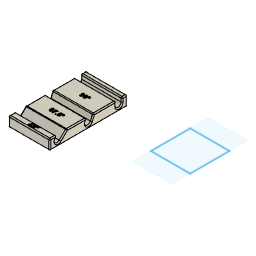
boulderStand v3 (Autodesk Fusion 360 design; units mm, degrees)
Autodesk Fusion 360 part; units mm, degrees
(part 1 of 3)
sketch "Sketch1" plane through (0, 0, 0) normal (0, 0, 1) x (1, 0, 0)
  line L0 (0, 0) -> (80, 0)
  line L1 (80, 0) -> (80, 150)
  line L2 (80, 150) -> (0, 150)
  line L3 (0, 150) -> (0, 0)
  dimension "d1" = 80
  dimension "d2" = 150
  constraint horizontal L0
  constraint vertical L1
  constraint horizontal L2
  constraint vertical L3
  constraint coincident L0.start L3.end
  measures "d1" distance of L0.start L0.end
  measures "d2" distance of L0.start L2.end
extrude "Extrude1" add sketch "Sketch1" along normal blind 20
sketch "Sketch2" plane through (0, 0, 0) normal (-1, 0, 0) x (0, -1, 0)
  line L0 (-150, 0) -> (0, 0)
  line L1 (0, 0) -> (0, 20)
  line L2 (0, 20) -> (-150, 20)
  line L3 (-150, 20) -> (-150, 0)
  line L4 (-140, 10) -> (-134, 10)
  arc A0 (-139.9709, 11.6408) -> (-127.9709, 11.6408) centre (-133.9709, 11.6408) ccw
  line L5 (-139.9709, 11.6408) -> (-139.9709, 20)
  line L6 (-127.9709, 11.6408) -> (-127.9709, 20)
  line L7 (-127.9709, 20) -> (-139.9709, 20)
  line L8 (-75, 20) -> (-127.9709, 20)
  arc A1 (-20.2732, 7.3711) -> (-11.8989, 15.9655) centre (-16.0578, 11.6408) ccw
  line L9 (-20.2732, 7.3711) -> (-33.0648, 20)
  line L10 (-11.8989, 15.9655) -> (-16.0943, 20)
  line L11 (0, 10) -> (-10, 10)
  circle A2 centre (-75, 11.6408) radius 6
  line L12 (-75, 11.6408) -> (-65.6617, 11.6408) construction
  line L13 (-80.5433, 9.3447) -> (-85.7662, 21.9539)
  line L14 (-69.4567, 13.9369) -> (-75, 27.3195)
  line L15 (-85.4501, 21.1908) -> (-74.3636, 25.783)
  dimension "d11" = 6
  dimension "d12" = 10
  dimension "d13" = 12
  constraint midpoint L1 L11.start
  constraint midpoint L2 L8.start
  constraint coincident L2 L5.end
  constraint tangent A0 L5
  constraint perpendicular L2 L5
  constraint coincident L2 L6.end
  constraint tangent A0 L6
  constraint perpendicular L2 L6
  constraint perpendicular L5 L7
  constraint coincident L2 L9.end
  constraint tangent A1 L9
  constraint coincident L2 L10.end
  constraint tangent A1 L10
  constraint perpendicular L1 L11
  constraint horizontal L12
  constraint coincident A2.centre L12.start
  constraint coincident A2 L14.start
  constraint coincident A2 L13.start
  constraint tangent A2 L13
  constraint tangent A2 L14
  constraint coincident L13 L15.start
  constraint coincident L14 L15.end
  constraint perpendicular L14 L15
  measures "d11" radius of A1
  measures "d12" distance of L11.start L11.end
  measures "d13" diameter of A2
extrude "Extrude2" cut sketch "Sketch2" against normal blind 113 contours L2 A0 L5 L6 L7 | L2 A1 L9 L10 | L2 L8 A2 L13 L14 | A2
fillet "Fillet1" radius 2 42 edges at (0, 0, 10) (40, 71.9682, 20) (80, 150, 10) (40, 150, 0) (0, 144.9854, 20) (80, 8.0471, 20) (80, 0, 10) (40, 150, 20) (40, 139.9709, 20) (0, 150, 10) (0, 75, 0) (0, 52.5165, 20) (80, 52.5165, 20) (80, 26.669, 13.6855) (80, 11.7605, 7.4535) (80, 13.9966, 17.9828) (80, 82.7501, 14.6723) (80, 72.7039, 6.0975) (80, 70.7124, 16.9684) (40, 0, 0) (80, 144.9854, 20) (0, 106.4639, 20) (0, 127.9709, 15.8204) (0, 133.9709, 5.6408) (0, 139.9709, 15.8204) (80, 75, 0) (0, 8.0471, 20) (0, 13.9966, 17.9828) (0, 11.7605, 7.4535) (0, 26.669, 13.6855) (0, 70.7124, 16.9684) (0, 72.7039, 6.0975) (0, 82.7501, 14.6723) (40, 127.9709, 20) (40, 0, 20) (80, 106.4639, 20) (80, 139.9709, 15.8204) (80, 133.9709, 5.6408) (80, 127.9709, 15.8204) (40, 33.0648, 20) (40, 16.0943, 20) (40, 84.9569, 20) 18 faces at (26.6667, 100, 0) (0, 41.0289, 12.0365) (80, 41.0289, 12.0365) (53.3333, 150, 6.6667) (53.3333, 69.3492, 13.6577) (26.6667, 82.0145, 12.8964) (26.6667, 70.2939, 15.9579) (26.6667, 13.2974, 17.3103) (53.3333, 11.5051, 15.5488) (53.3333, 24.5371, 11.5807) (26.6667, 0, 6.6667) (26.6667, 146.657, 20) (53.3333, 46.0326, 20) (26.6667, 127.9709, 14.4272) (53.3333, 135.8818, 5.9532) (26.6667, 139.9709, 14.4272) (26.6667, 10.7295, 20) (26.6667, 113.6329, 20)
sketch "Sketch3" plane through (0, 0, 20) normal (0, 0, 1) x (-1, 0, 0)
  line L0 (-2, -2) -> (-78, -2)
  line L1 (-78, -2) -> (-78, -11.1292)
  line L2 (-78, -11.1292) -> (-2, -11.1292)
  line L3 (-2, -11.1292) -> (-2, -2)
  line L4 (-2, -2) -> (-78, -2) construction
  line L5 (-78, -2) -> (-78, -11.1292) construction
  line L6 (-78, -11.1292) -> (-2, -11.1292) construction
  line L7 (-2, -11.1292) -> (-2, -2) construction
  dimension "d21" = 8
  text T0 "45" font "Arial" height 8 bold align centre middle in box 76 x 9.1292 at (-2, -2) x (-1, 0) y (0, -1) spacing 1
  constraint coincident L0.end
  constraint coincident L2.end
sketch "Sketch4" plane through (0, 0, 20) normal (0, 0, 1) x (-1, 0, 0)
  line L0 (-78, -33.8858) -> (-78, -68.9749)
  line L1 (-78, -68.9749) -> (-2, -68.9749)
  line L2 (-2, -68.9749) -> (-2, -33.8858)
  line L3 (-2, -33.8858) -> (-78, -33.8858)
  line L4 (-2, -33.8858) -> (-78, -33.8858) construction
  line L5 (-78, -33.8858) -> (-78, -68.9749) construction
  line L6 (-78, -68.9749) -> (-2, -68.9749) construction
  line L7 (-2, -68.9749) -> (-2, -33.8858) construction
  line L8 (-50.8421, -33.8858) -> (-58.1757, -33.8858) construction
  line L9 (-58.1757, -33.8858) -> (-58.1757, -68.9749) construction
  line L10 (-58.1757, -68.9749) -> (-50.8421, -68.9749) construction
  line L11 (-50.8421, -68.9749) -> (-50.8421, -33.8858) construction
  dimension "d22" = 8
  dimension "d25" = 8
  text T0 "67.5" font "Arial" height 8 bold align centre middle in box 76 x 35.0892 at (-2, -33.8858) x (-1, 0) y (0, -1) spacing 1
  text T1 "°" font "Arial" height 8 bold align left middle in box 7.3337 x 35.0892 at (-50.8421, -33.8858) x (-1, 0) y (0, -1) spacing 1
  constraint coincident L0.start
  constraint coincident L1.end
  constraint coincident L3
  constraint coincident L1
sketch "Sketch5" plane through (0, 0, 20) normal (0, 0, 1) x (1, 0, 0)
  line L0 (46.54, 2) -> (52.8374, 2) construction
  line L1 (52.8374, 2) -> (52.8374, 11.1292) construction
  line L2 (52.8374, 11.1292) -> (46.54, 11.1292) construction
  line L3 (46.54, 11.1292) -> (46.54, 2) construction
  line L4 (78, 11.1292) -> (2, 11.1292)
  line L5 (2, 2) -> (78, 2)
  dimension "d24" = 8
  text T0 "°" font "Arial" height 8 bold align left middle in box 6.2975 x 9.1292 at (46.54, 2) x (1, 0) y (0, 1) spacing 1
  constraint coincident L5
  constraint coincident L4
sketch "Sketch6" plane through (0, 0, 20) normal (0, 0, 1) x (-1, 0, 0)
  line L0 (-2, -125.9709) -> (-2, -86.2932)
  line L1 (-2, -86.2932) -> (-78, -86.2932)
  line L2 (-78, -86.2932) -> (-78, -125.9709)
  line L3 (-78, -125.9709) -> (-2, -125.9709)
  line L4 (-2, -86.2932) -> (-78, -86.2932) construction
  line L5 (-78, -86.2932) -> (-78, -125.9709) construction
  line L6 (-78, -125.9709) -> (-2, -125.9709) construction
  line L7 (-2, -125.9709) -> (-2, -86.2932) construction
  line L8 (-46.334, -86.2932) -> (-50.8421, -86.2932) construction
  line L9 (-50.8421, -86.2932) -> (-50.8421, -125.9709) construction
  line L10 (-50.8421, -125.9709) -> (-46.334, -125.9709) construction
  line L11 (-46.334, -125.9709) -> (-46.334, -86.2932) construction
  dimension "d26" = 8
  dimension "d27" = 8
  text T0 "90" font "Arial" height 8 bold align centre middle in box 76 x 39.6776 at (-2, -86.2932) x (-1, 0) y (0, -1) spacing 1
  text T1 "°" font "Arial" height 8 bold align left middle in box 4.5081 x 39.6776 at (-46.334, -86.2932) x (-1, 0) y (0, -1) spacing 1
  constraint coincident L1.end
  constraint coincident L0.start
  constraint coincident L1
  constraint coincident L3
extrude "Extrude3" cut sketch "Sketch6" sketch "Sketch3" sketch "Sketch5" sketch "Sketch4" against normal blind 5 text T1 T0 of sketch 2 text T0 of sketch 3 text T0 of sketch 4 text T1 T0
sketch "Sketch7" plane through (0, 0, 20) normal (0, 0, 1) x (-1, 0, 0)
  line L0 (-2, -141.9709) -> (-78, -141.9709)
  line L1 (-78, -141.9709) -> (-78, -148)
  line L2 (-78, -148) -> (-2, -148)
  line L3 (-2, -148) -> (-2, -141.9709)
  line L4 (-2, -141.9709) -> (-78, -141.9709) construction
  line L5 (-78, -141.9709) -> (-78, -148) construction
  line L6 (-78, -148) -> (-2, -148) construction
  line L7 (-2, -148) -> (-2, -141.9709) construction
  line L8 (-53.7035, -144.1937) -> (-57.3792, -144.1937) construction
  line L9 (-57.3792, -144.1937) -> (-57.3792, -147.5652) construction
  line L10 (-57.3792, -147.5652) -> (-53.7035, -147.5652) construction
  line L11 (-53.7035, -147.5652) -> (-53.7035, -144.1937) construction
  dimension "d30" = 3
  dimension "d31" = 2
  text T0 "boulderStand" font "Arial" height 3 bold align centre middle in box 76 x 6.0291 at (-2, -141.9709) x (-1, 0) y (0, -1) spacing 1
  text T1 "™" font "Arial" height 2 bold align left top in box 3.6757 x 3.3715 at (-53.7035, -144.1937) x (-1, 0) y (0, -1) spacing 1
  constraint coincident L0.end
  constraint coincident L2.end
extrude "Extrude4" cut sketch "Sketch7" against normal blind 5 text T1 T0
extrude "Extrude5" cut 1 faces at (10.2557, 145.4854, 20) along direction (0, 0, -1) blind 5
extrude "Extrude6" add 1 faces at (10.446, 144.8633, 15) along direction (0, 0, 1) blind 5
sketch "Sketch8" plane through (0, 0, 0) normal (0, 0, -1) x (1, 0, 0)
  line L0 (2, -2) -> (2, -148)
  line L1 (2, -148) -> (78, -148)
  line L2 (78, -148) -> (78, -2)
  line L3 (78, -2) -> (2, -2)
  line L4 (78, -148) -> (78, -2) construction
  line L5 (78, -2) -> (2, -2) construction
  line L6 (2, -2) -> (2, -148) construction
  line L7 (2, -148) -> (78, -148) construction
  dimension "d38" = 10
  constraint coincident L2.end
  constraint coincident L0.end
sketch "Sketch9" plane through (0, 0, 0) normal (0, 0, -1) x (1, 0, 0)
  line L0 (2, -2) -> (2, -148)
  line L1 (2, -148) -> (78, -148)
  line L2 (78, -148) -> (78, -2)
  line L3 (78, -2) -> (2, -2)
  line L4 (2, -113) -> (78, -113)
  line L5 (78, -113) -> (78, -37)
  line L6 (78, -37) -> (2, -37)
  line L7 (2, -37) -> (2, -113)
  dimension "d41" = 76
  dimension "d42" = 76
  constraint horizontal L4
  constraint vertical L5
  constraint horizontal L6
  constraint vertical L7
  measures "d41" distance of L4.start L4.end
  measures "d42" distance of L4.start L6.end
move_body "Move1" bodies 1 to x (1, 0, 0) y (0, 1, 0) z (0, 0, 1) at (-78, -113, 0)
sketch "Sketch11" plane through (0, 0, 0) normal (0, 0, -1) x (1, 0, 0)
  line L0 (-76, 111) -> (-76, -35)
  line L1 (-76, -35) -> (0, -35)
  line L2 (0, -35) -> (0, 111)
  line L3 (0, 111) -> (-76, 111)
  spline S0 degree 3 poles (-138.6954, -42.4873) (-137.8482, -42.938) (-137.0232, -43.3505) (-136.2275, -43.8133) knots 0 0 0 0 1 1 1 1
  spline S1 degree 3 poles (-136.2275, -43.8133) (-135.8004, -44.0617) (-135.4472, -44.0483) (-135.0165, -43.8171) knots 0 0 0 0 1 1 1 1
  spline S2 degree 3 poles (-135.0165, -43.8171) (-130.9901, -41.6554) (-126.96, -39.5003) (-122.9201, -37.3639) knots 0 0 0 0 1 1 1 1
  spline S3 degree 3 poles (-122.9201, -37.3639) (-117.1136, -34.2933) (-111.3019, -31.2326) (-105.4798, -28.1918) knots 0 0 0 0 1 1 1 1
  spline S4 degree 3 poles (-105.4798, -28.1918) (-104.9534, -27.9169) (-104.7523, -27.6043) (-104.7927, -27.0205) knots 0 0 0 0 1 1 1 1
  spline S5 degree 3 poles (-104.7927, -27.0205) (-104.8438, -26.2818) (-104.805, -25.5368) (-104.805, -24.8271) knots 0 0 0 0 1 1 1 1
  spline S6 degree 3 poles (-104.805, -24.8271) (-105.0619, -24.7236) (-105.1888, -24.8414) (-105.3223, -24.9086) knots 0 0 0 0 1 1 1 1
  spline S7 degree 3 poles (-105.3223, -24.9086) (-110.8488, -27.6894) (-116.3746, -30.4718) (-121.8995, -33.2557) knots 0 0 0 0 1 1 1 1
  spline S8 degree 3 poles (-121.8995, -33.2557) (-124.5222, -34.5772) (-127.1429, -35.9024) (-129.7648, -37.2253) knots 0 0 0 0 1 1 1 1
  spline S9 degree 3 poles (-129.7648, -37.2253) (-129.8579, -37.2722) (-129.9526, -37.3166) (-130.0492, -37.3554) knots 0 0 0 0 1 1 1 1
  spline S10 degree 3 poles (-130.0492, -37.3554) (-130.2324, -37.4291) (-130.4258, -37.493) (-130.5657, -37.2915) knots 0 0 0 0 1 1 1 1
  spline S11 degree 3 poles (-130.5657, -37.2915) (-130.6846, -37.1204) (-130.6008, -36.9572) (-130.492, -36.8125) knots 0 0 0 0 1 1 1 1
  spline S12 degree 3 poles (-130.492, -36.8125) (-130.095, -36.2847) (-129.7039, -35.7521) (-129.2948, -35.2338) knots 0 0 0 0 1 1 1 1
  spline S13 degree 3 poles (-129.2948, -35.2338) (-127.8735, -33.4331) (-126.4152, -31.6629) (-124.9238, -29.9195) knots 0 0 0 0 1 1 1 1
  spline S14 degree 3 poles (-124.9238, -29.9195) (-124.7073, -29.6665) (-124.5263, -29.6417) (-124.2573, -29.7965) knots 0 0 0 0 1 1 1 1
  spline S15 degree 3 poles (-124.2573, -29.7965) (-123.7452, -30.091) (-123.2141, -30.3533) (-122.7096, -30.6598) knots 0 0 0 0 1 1 1 1
  spline S16 degree 3 poles (-122.7096, -30.6598) (-122.3871, -30.8558) (-122.1406, -30.858) (-121.8247, -30.6176) knots 0 0 0 0 1 1 1 1
  spline S17 degree 3 poles (-121.8247, -30.6176) (-119.5704, -28.9025) (-117.3017, -27.2063) (-115.0379, -25.5036) knots 0 0 0 0 1 1 1 1
  spline S18 degree 3 poles (-115.0379, -25.5036) (-113.4546, -24.3128) (-111.8622, -23.1339) (-110.2938, -21.9237) knots 0 0 0 0 1 1 1 1
  spline S19 degree 3 poles (-110.2938, -21.9237) (-109.6956, -21.4621) (-109.1101, -21.2309) (-108.3057, -21.2604) knots 0 0 0 0 1 1 1 1
  spline S20 degree 3 poles (-108.3057, -21.2604) (-106.0485, -21.343) (-103.7864, -21.2881) (-101.5262, -21.2879) knots 0 0 0 0 1 1 1 1
  spline S21 degree 3 poles (-101.5262, -21.2879) (-100.7062, -21.2878) (-100.7051, -21.2884) (-100.7048, -22.1146) knots 0 0 0 0 1 1 1 1
  spline S22 degree 3 poles (-100.7048, -22.1146) (-100.7041, -24.7051) (-100.7139, -27.2957) (-100.6947, -29.8861) knots 0 0 0 0 1 1 1 1
  spline S23 degree 3 poles (-100.6947, -29.8861) (-100.6915, -30.3254) (-100.8261, -30.5762) (-101.221, -30.7832) knots 0 0 0 0 1 1 1 1
  spline S24 degree 3 poles (-101.221, -30.7832) (-105.7621, -33.1626) (-110.2947, -35.5582) (-114.8293, -37.9501) knots 0 0 0 0 1 1 1 1
  spline S25 degree 3 poles (-114.8293, -37.9501) (-119.7786, -40.5607) (-124.7257, -43.1757) (-129.6778, -45.781) knots 0 0 0 0 1 1 1 1
  spline S26 degree 3 poles (-129.6778, -45.781) (-131.4926, -46.7358) (-133.3237, -47.6594) (-135.1361, -48.6183) knots 0 0 0 0 1 1 1 1
  spline S27 degree 3 poles (-135.1361, -48.6183) (-135.501, -48.8114) (-135.7908, -48.8066) (-136.1538, -48.6139) knots 0 0 0 0 1 1 1 1
  spline S28 degree 3 poles (-136.1538, -48.6139) (-141.2502, -45.9094) (-146.3535, -43.2181) (-151.4549, -40.5231) knots 0 0 0 0 1 1 1 1
  spline S29 degree 3 poles (-151.4549, -40.5231) (-156.7716, -37.7144) (-162.0881, -34.9056) (-167.4041, -32.0956) knots 0 0 0 0 1 1 1 1
  spline S30 degree 3 poles (-167.4041, -32.0956) (-168.2645, -31.6408) (-169.1167, -31.1702) (-169.9826, -30.7264) knots 0 0 0 0 1 1 1 1
  spline S31 degree 3 poles (-169.9826, -30.7264) (-170.3174, -30.5548) (-170.454, -30.3268) (-170.4526, -29.9451) knots 0 0 0 0 1 1 1 1
  spline S32 degree 3 poles (-170.4526, -29.9451) (-170.4425, -27.2329) (-170.4425, -24.5206) (-170.4611, -21.8085) knots 0 0 0 0 1 1 1 1
  spline S33 degree 3 poles (-170.4611, -21.8085) (-170.4641, -21.362) (-170.2794, -21.2348) (-169.8758, -21.2352) knots 0 0 0 0 1 1 1 1
  spline S34 degree 3 poles (-169.8758, -21.2352) (-165.1989, -21.2398) (-160.5221, -21.238) (-155.8453, -21.2375) knots 0 0 0 0 1 1 1 1
  spline S35 degree 3 poles (-155.8453, -21.2375) (-155.5971, -21.2374) (-155.3642, -21.2992) (-155.1393, -21.399) knots 0 0 0 0 1 1 1 1
  spline S36 degree 3 poles (-155.1393, -21.399) (-154.7263, -21.5823) (-154.3289, -21.8305) (-153.8968, -21.9352) knots 0 0 0 0 1 1 1 1
  spline S37 degree 3 poles (-153.8968, -21.9352) (-152.5328, -22.2658) (-151.9591, -23.261) (-151.5082, -24.4698) knots 0 0 0 0 1 1 1 1
  spline S38 degree 3 poles (-151.5082, -24.4698) (-150.8226, -26.308) (-150.0383, -28.1095) (-149.2921, -29.9249) knots 0 0 0 0 1 1 1 1
  spline S39 degree 3 poles (-149.2921, -29.9249) (-149.0409, -30.5359) (-149.0115, -30.5499) (-148.4317, -30.2451) knots 0 0 0 0 1 1 1 1
  spline S40 degree 3 poles (-148.4317, -30.2451) (-147.9552, -29.9946) (-147.4824, -29.7341) (-147.0257, -29.4496) knots 0 0 0 0 1 1 1 1
  spline S41 degree 3 poles (-147.0257, -29.4496) (-146.7529, -29.2797) (-146.5802, -29.2895) (-146.3723, -29.558) knots 0 0 0 0 1 1 1 1
  spline S42 degree 3 poles (-146.3723, -29.558) (-144.6811, -31.7435) (-142.9733, -33.9162) (-141.2815, -36.1012) knots 0 0 0 0 1 1 1 1
  spline S43 degree 3 poles (-141.2815, -36.1012) (-140.9996, -36.4653) (-140.6833, -36.8234) (-140.5966, -37.324) knots 0 0 0 0 1 1 1 1
  spline S44 degree 3 poles (-140.5966, -37.324) (-140.9781, -37.5612) (-141.281, -37.3359) (-141.5728, -37.1854) knots 0 0 0 0 1 1 1 1
  spline S45 degree 3 poles (-141.5728, -37.1854) (-143.4107, -36.2375) (-145.2363, -35.2657) (-147.0775, -34.3242) knots 0 0 0 0 1 1 1 1
  spline S46 degree 3 poles (-147.0775, -34.3242) (-150.2955, -32.6787) (-153.5196, -31.0448) (-156.7454, -29.4145) knots 0 0 0 0 1 1 1 1
  spline S47 degree 3 poles (-156.7454, -29.4145) (-159.7388, -27.9017) (-162.7377, -26.3998) (-165.7346, -24.8937) knots 0 0 0 0 1 1 1 1
  spline S48 degree 3 poles (-165.7346, -24.8937) (-165.8884, -24.8163) (-166.0451, -24.7446) (-166.2362, -24.6531) knots 0 0 0 0 1 1 1 1
  spline S49 degree 3 poles (-166.2362, -24.6531) (-166.4023, -25.0969) (-166.2477, -25.5363) (-166.3286, -25.9459) knots 0 0 0 0 1 1 1 1
  spline S50 degree 3 poles (-166.3286, -25.9459) (-166.6138, -27.3907) (-165.9303, -28.0763) (-164.6637, -28.7299) knots 0 0 0 0 1 1 1 1
  spline S51 degree 3 poles (-164.6637, -28.7299) (-157.9466, -32.1962) (-151.2881, -35.7762) (-144.6115, -39.3209) knots 0 0 0 0 1 1 1 1
  spline S52 degree 3 poles (-144.6115, -39.3209) (-142.6473, -40.3637) (-140.6902, -41.42) (-138.6954, -42.4873) knots 0 0 0 0 1 1 1 1
  spline S53 degree 3 poles (-167.2917, -4.2439) (-168.1435, -4.2459) (-168.9433, -4.2401) (-169.7428, -4.2527) knots 0 0 0 0 1 1 1 1
  spline S54 degree 3 poles (-169.7428, -4.2527) (-170.2186, -4.2602) (-170.4461, -4.0604) (-170.4449, -3.5707) knots 0 0 0 0 1 1 1 1
  spline S55 degree 3 poles (-170.4449, -3.5707) (-170.44, -1.4847) (-170.4414, 0.6014) (-170.4549, 2.6874) knots 0 0 0 0 1 1 1 1
  spline S56 degree 3 poles (-170.4549, 2.6874) (-170.4573, 3.0554) (-170.2378, 3.2021) (-169.9645, 3.3442) knots 0 0 0 0 1 1 1 1
  spline S57 degree 3 poles (-169.9645, 3.3442) (-165.0165, 5.9171) (-160.0627, 8.479) (-155.1245, 11.0703) knots 0 0 0 0 1 1 1 1
  spline S58 degree 3 poles (-155.1245, 11.0703) (-148.7857, 14.3966) (-142.4581, 17.7442) (-136.1317, 21.0941) knots 0 0 0 0 1 1 1 1
  spline S59 degree 3 poles (-136.1317, 21.0941) (-135.7867, 21.2768) (-135.5231, 21.2875) (-135.1713, 21.1037) knots 0 0 0 0 1 1 1 1
  spline S60 degree 3 poles (-135.1713, 21.1037) (-126.7014, 16.6786) (-118.2257, 12.2644) (-109.7495, 7.8514) knots 0 0 0 0 1 1 1 1
  spline S61 degree 3 poles (-109.7495, 7.8514) (-106.9139, 6.3751) (-104.0771, 4.9011) (-101.2318, 3.4438) knots 0 0 0 0 1 1 1 1
  spline S62 degree 3 poles (-101.2318, 3.4438) (-100.8569, 3.2517) (-100.6975, 3.0249) (-100.7012, 2.5987) knots 0 0 0 0 1 1 1 1
  spline S63 degree 3 poles (-100.7012, 2.5987) (-100.7185, 0.5823) (-100.7063, -1.4343) (-100.7098, -3.4508) knots 0 0 0 0 1 1 1 1
  spline S64 degree 3 poles (-100.7098, -3.4508) (-100.7109, -4.0585) (-100.8717, -4.239) (-101.4803, -4.2403) knots 0 0 0 0 1 1 1 1
  spline S65 degree 3 poles (-101.4803, -4.2403) (-105.7567, -4.2497) (-110.0332, -4.2518) (-114.3096, -4.2476) knots 0 0 0 0 1 1 1 1
  spline S66 degree 3 poles (-114.3096, -4.2476) (-114.9414, -4.247) (-114.9961, -4.1356) (-114.994, -3.5028) knots 0 0 0 0 1 1 1 1
  spline S67 degree 3 poles (-114.994, -3.5028) (-114.9885, -1.8522) (-115.0102, -0.2014) (-115.0183, 1.4493) knots 0 0 0 0 1 1 1 1
  spline S68 degree 3 poles (-115.0183, 1.4493) (-115.0192, 1.6365) (-115.0544, 1.8329) (-114.9008, 2.034) knots 0 0 0 0 1 1 1 1
  spline S69 degree 3 poles (-114.9008, 2.034) (-114.6084, 2.0558) (-114.3671, 1.8698) (-114.1154, 1.739) knots 0 0 0 0 1 1 1 1
  spline S70 degree 3 poles (-114.1154, 1.739) (-112.3576, 0.826) (-110.598, -0.084) (-108.8524, -1.0199) knots 0 0 0 0 1 1 1 1
  spline S71 degree 3 poles (-108.8524, -1.0199) (-108.4238, -1.2496) (-108.0662, -1.255) (-107.6381, -1.0212) knots 0 0 0 0 1 1 1 1
  spline S72 degree 3 poles (-107.6381, -1.0212) (-106.7737, -0.5493) (-105.8835, -0.125) (-104.9491, 0.3466) knots 0 0 0 0 1 1 1 1
  spline S73 degree 3 poles (-104.9491, 0.3466) (-105.2471, 0.6307) (-105.5649, 0.769) (-105.8649, 0.925) knots 0 0 0 0 1 1 1 1
  spline S74 degree 3 poles (-105.8649, 0.925) (-112.2933, 4.2675) (-118.7283, 7.5976) (-125.1523, 10.9486) knots 0 0 0 0 1 1 1 1
  spline S75 degree 3 poles (-125.1523, 10.9486) (-128.5107, 12.7005) (-131.8525, 14.4844) (-135.1958, 16.2651) knots 0 0 0 0 1 1 1 1
  spline S76 degree 3 poles (-135.1958, 16.2651) (-135.5025, 16.4284) (-135.7414, 16.4451) (-136.0596, 16.2762) knots 0 0 0 0 1 1 1 1
  spline S77 degree 3 poles (-136.0596, 16.2762) (-143.8411, 12.1461) (-151.6057, 7.9841) (-159.4381, 3.9505) knots 0 0 0 0 1 1 1 1
  spline S78 degree 3 poles (-159.4381, 3.9505) (-161.6009, 2.8367) (-163.7552, 1.7064) (-165.9128, 0.5824) knots 0 0 0 0 1 1 1 1
  spline S79 degree 3 poles (-165.9128, 0.5824) (-166.0183, 0.5275) (-166.1172, 0.46) (-166.2911, 0.3548) knots 0 0 0 0 1 1 1 1
  spline S80 degree 3 poles (-166.2911, 0.3548) (-165.2018, -0.1905) (-164.1707, -0.7085) (-163.1376, -1.2224) knots 0 0 0 0 1 1 1 1
  spline S81 degree 3 poles (-163.1376, -1.2224) (-162.8737, -1.3537) (-162.6696, -1.1739) (-162.4598, -1.0643) knots 0 0 0 0 1 1 1 1
  spline S82 degree 3 poles (-162.4598, -1.0643) (-160.7503, -0.1715) (-159.0445, 0.7284) (-157.3335, 1.6183) knots 0 0 0 0 1 1 1 1
  spline S83 degree 3 poles (-157.3335, 1.6183) (-157.015, 1.7839) (-156.703, 1.9776) (-156.3451, 2.0338) knots 0 0 0 0 1 1 1 1
  spline S84 degree 3 poles (-156.3451, 2.0338) (-156.1446, 1.8753) (-156.2021, 1.6696) (-156.2016, 1.4897) knots 0 0 0 0 1 1 1 1
  spline S85 degree 3 poles (-156.2016, 1.4897) (-156.1967, -0.2139) (-156.2165, -1.9178) (-156.1893, -3.621) knots 0 0 0 0 1 1 1 1
  spline S86 degree 3 poles (-156.1893, -3.621) (-156.181, -4.1429) (-156.3819, -4.2618) (-156.8618, -4.2594) knots 0 0 0 0 1 1 1 1
  spline S87 degree 3 poles (-156.8618, -4.2594) (-160.321, -4.2416) (-163.7803, -4.2463) (-167.2917, -4.2439) knots 0 0 0 0 1 1 1 1
  spline S88 degree 3 poles (-129.5885, -30.8645) (-131.3563, -33.0127) (-133.0918, -35.139) (-134.8483, -37.2477) knots 0 0 0 0 1 1 1 1
  spline S89 degree 3 poles (-134.8483, -37.2477) (-135.5907, -38.139) (-135.7378, -38.1243) (-136.4614, -37.2414) knots 0 0 0 0 1 1 1 1
  spline S90 degree 3 poles (-136.4614, -37.2414) (-140.0179, -32.902) (-143.5716, -28.5603) (-147.1288, -24.2216) knots 0 0 0 0 1 1 1 1
  spline S91 degree 3 poles (-147.1288, -24.2216) (-147.7785, -23.429) (-148.4426, -22.6483) (-149.0934, -21.8567) knots 0 0 0 0 1 1 1 1
  spline S92 degree 3 poles (-149.0934, -21.8567) (-149.211, -21.7136) (-149.3661, -21.5851) (-149.3959, -21.2442) knots 0 0 0 0 1 1 1 1
  spline S93 degree 3 poles (-149.3959, -21.2442) (-148.8253, -21.2442) (-148.2643, -21.2392) (-147.7034, -21.2452) knots 0 0 0 0 1 1 1 1
  spline S94 degree 3 poles (-147.7034, -21.2452) (-146.7134, -21.2558) (-145.7234, -21.2874) (-144.7336, -21.2801) knots 0 0 0 0 1 1 1 1
  spline S95 degree 3 poles (-144.7336, -21.2801) (-144.3687, -21.2774) (-144.1071, -21.4064) (-143.8691, -21.6648) knots 0 0 0 0 1 1 1 1
  spline S96 degree 3 poles (-143.8691, -21.6648) (-141.292, -24.4631) (-138.7102, -27.2571) (-136.1313, -30.0538) knots 0 0 0 0 1 1 1 1
  spline S97 degree 3 poles (-136.1313, -30.0538) (-135.7138, -30.5065) (-135.6981, -30.5094) (-135.2613, -30.0386) knots 0 0 0 0 1 1 1 1
  spline S98 degree 3 poles (-135.2613, -30.0386) (-132.651, -27.2246) (-130.0396, -24.4116) (-127.4317, -21.5953) knots 0 0 0 0 1 1 1 1
  spline S99 degree 3 poles (-127.4317, -21.5953) (-127.2331, -21.3808) (-127.0179, -21.238) (-126.7128, -21.2386) knots 0 0 0 0 1 1 1 1
  spline S100 degree 3 poles (-126.7128, -21.2386) (-125.2184, -21.2415) (-123.724, -21.2367) (-122.2297, -21.2379) knots 0 0 0 0 1 1 1 1
  spline S101 degree 3 poles (-122.2297, -21.2379) (-122.0945, -21.238) (-121.9467, -21.2209) (-121.7959, -21.4251) knots 0 0 0 0 1 1 1 1
  spline S102 degree 3 poles (-121.7959, -21.4251) (-124.3764, -24.5509) (-126.9706, -27.6932) (-129.5885, -30.8645) knots 0 0 0 0 1 1 1 1
  spline S103 degree 3 poles (-133.3885, 6.0697) (-138.1944, 6.0697) (-142.9482, 6.0697) (-147.704, 6.0697) knots 0 0 0 0 1 1 1 1
  spline S104 degree 3 poles (-147.704, 6.0697) (-147.7334, 6.4091) (-147.5064, 6.4516) (-147.3578, 6.5361) knots 0 0 0 0 1 1 1 1
  spline S105 degree 3 poles (-147.3578, 6.5361) (-143.6579, 8.6387) (-139.9086, 10.6502) (-136.1468, 12.6393) knots 0 0 0 0 1 1 1 1
  spline S106 degree 3 poles (-136.1468, 12.6393) (-135.7511, 12.8485) (-135.4346, 12.8423) (-135.0354, 12.6282) knots 0 0 0 0 1 1 1 1
  spline S107 degree 3 poles (-135.0354, 12.6282) (-131.301, 10.6256) (-127.5551, 8.6445) (-123.8144, 6.6534) knots 0 0 0 0 1 1 1 1
  spline S108 degree 3 poles (-123.8144, 6.6534) (-123.6231, 6.5516) (-123.389, 6.4826) (-123.2929, 6.0698) knots 0 0 0 0 1 1 1 1
  spline S109 degree 3 poles (-123.2929, 6.0698) (-126.6676, 6.0698) (-130.002, 6.0698) (-133.3885, 6.0697) knots 0 0 0 0 1 1 1 1
  spline S110 degree 3 poles (-111.1725, -8.9308) (-110.5209, -8.0007) (-109.6558, -7.6048) (-108.562, -7.6257) knots 0 0 0 0 1 1 1 1
  spline S111 degree 3 poles (-108.562, -7.6257) (-107.2938, -7.65) (-106.0245, -7.6481) (-104.7564, -7.6236) knots 0 0 0 0 1 1 1 1
  spline S112 degree 3 poles (-104.7564, -7.6236) (-104.2958, -7.6147) (-104.1568, -7.7765) (-104.1597, -8.2273) knots 0 0 0 0 1 1 1 1
  spline S113 degree 3 poles (-104.1597, -8.2273) (-104.1795, -11.2683) (-104.1769, -14.3095) (-104.1833, -17.3506) knots 0 0 0 0 1 1 1 1
  spline S114 degree 3 poles (-104.1833, -17.3506) (-104.1839, -17.6258) (-104.1355, -17.9474) (-104.5726, -17.9266) knots 0 0 0 0 1 1 1 1
  spline S115 degree 3 poles (-104.5726, -17.9266) (-106.152, -17.8511) (-107.7312, -18.102) (-109.3105, -17.9262) knots 0 0 0 0 1 1 1 1
  spline S116 degree 3 poles (-109.3105, -17.9262) (-110.6894, -17.7727) (-111.875, -16.1642) (-111.6746, -14.791) knots 0 0 0 0 1 1 1 1
  spline S117 degree 3 poles (-111.6746, -14.791) (-111.5769, -14.1209) (-111.4055, -13.4977) (-110.9836, -12.9696) knots 0 0 0 0 1 1 1 1
  spline S118 degree 3 poles (-110.9836, -12.9696) (-110.7848, -12.7208) (-110.9107, -12.5646) (-111.0475, -12.3778) knots 0 0 0 0 1 1 1 1
  spline S119 degree 3 poles (-111.0475, -12.3778) (-111.8568, -11.2727) (-111.849, -10.1313) (-111.1725, -8.9308) knots 0 0 0 0 1 1 1 1
  spline S120 degree 3 poles (-107.867, -13.6405) (-107.9879, -13.6413) (-108.1093, -13.6359) (-108.2297, -13.644) knots 0 0 0 0 1 1 1 1
  spline S121 degree 3 poles (-108.2297, -13.644) (-108.8642, -13.6864) (-109.266, -14.1021) (-109.2621, -14.7076) knots 0 0 0 0 1 1 1 1
  spline S122 degree 3 poles (-109.2621, -14.7076) (-109.2584, -15.2831) (-108.8634, -15.6362) (-108.1995, -15.6527) knots 0 0 0 0 1 1 1 1
  spline S123 degree 3 poles (-108.1995, -15.6527) (-107.975, -15.6583) (-107.7502, -15.6556) (-107.5256, -15.6558) knots 0 0 0 0 1 1 1 1
  spline S124 degree 3 poles (-107.5256, -15.6558) (-106.7257, -15.6565) (-106.7257, -15.6564) (-106.6728, -14.8445) knots 0 0 0 0 1 1 1 1
  spline S125 degree 3 poles (-106.6728, -14.8445) (-106.5945, -13.643) (-106.5945, -13.643) (-107.867, -13.6405) knots 0 0 0 0 1 1 1 1
  spline S126 degree 3 poles (-109.251, -10.5792) (-109.23, -11.2221) (-108.9751, -11.4906) (-108.3471, -11.5248) knots 0 0 0 0 1 1 1 1
  spline S127 degree 3 poles (-108.3471, -11.5248) (-107.9675, -11.5454) (-107.5878, -11.5645) (-107.2078, -11.5766) knots 0 0 0 0 1 1 1 1
  spline S128 degree 3 poles (-107.2078, -11.5766) (-106.883, -11.587) (-106.6793, -11.4699) (-106.6896, -11.0975) knots 0 0 0 0 1 1 1 1
  spline S129 degree 3 poles (-106.6896, -11.0975) (-106.7287, -9.6896) (-106.408, -9.8232) (-107.9214, -9.8006) knots 0 0 0 0 1 1 1 1
  spline S130 degree 3 poles (-107.9214, -9.8006) (-108.0079, -9.7993) (-108.0951, -9.7925) (-108.1807, -9.8011) knots 0 0 0 0 1 1 1 1
  spline S131 degree 3 poles (-108.1807, -9.8011) (-108.6554, -9.8487) (-109.0535, -10.0152) (-109.251, -10.5792) knots 0 0 0 0 1 1 1 1
  spline S132 degree 3 poles (-159.1234, -14.4458) (-159.1237, -15.4706) (-159.1354, -16.4435) (-159.1189, -17.4158) knots 0 0 0 0 1 1 1 1
  spline S133 degree 3 poles (-159.1189, -17.4158) (-159.1124, -17.7976) (-159.2559, -17.9395) (-159.6354, -17.9359) knots 0 0 0 0 1 1 1 1
  spline S134 degree 3 poles (-159.6354, -17.9359) (-160.9031, -17.9241) (-162.1714, -17.953) (-163.4388, -17.9296) knots 0 0 0 0 1 1 1 1
  spline S135 degree 3 poles (-163.4388, -17.9296) (-164.9362, -17.902) (-166.2925, -16.5065) (-166.3951, -15.0074) knots 0 0 0 0 1 1 1 1
  spline S136 degree 3 poles (-166.3951, -15.0074) (-166.4909, -13.608) (-166.1705, -12.4241) (-164.9192, -11.6328) knots 0 0 0 0 1 1 1 1
  spline S137 degree 3 poles (-164.9192, -11.6328) (-164.72, -11.5069) (-164.7367, -11.3588) (-164.8353, -11.1911) knots 0 0 0 0 1 1 1 1
  spline S138 degree 3 poles (-164.8353, -11.1911) (-164.9233, -11.0416) (-165.0497, -10.9088) (-165.1102, -10.7499) knots 0 0 0 0 1 1 1 1
  spline S139 degree 3 poles (-165.1102, -10.7499) (-165.3877, -10.0212) (-165.9093, -9.7619) (-166.6581, -9.8998) knots 0 0 0 0 1 1 1 1
  spline S140 degree 3 poles (-166.6581, -9.8998) (-167.1168, -9.9843) (-167.2886, -9.7983) (-167.2438, -9.3302) knots 0 0 0 0 1 1 1 1
  spline S141 degree 3 poles (-167.2438, -9.3302) (-167.2043, -8.9169) (-167.2221, -8.4971) (-167.2311, -8.0805) knots 0 0 0 0 1 1 1 1
  spline S142 degree 3 poles (-167.2311, -8.0805) (-167.2374, -7.7908) (-167.1018, -7.6655) (-166.8261, -7.6675) knots 0 0 0 0 1 1 1 1
  spline S143 degree 3 poles (-166.8261, -7.6675) (-166.288, -7.6714) (-165.7498, -7.6706) (-165.2119, -7.6838) knots 0 0 0 0 1 1 1 1
  spline S144 degree 3 poles (-165.2119, -7.6838) (-164.4343, -7.7028) (-164.0029, -8.2235) (-163.6345, -8.8124) knots 0 0 0 0 1 1 1 1
  spline S145 degree 3 poles (-163.6345, -8.8124) (-163.2571, -9.4158) (-162.8892, -10.0257) (-162.5373, -10.6443) knots 0 0 0 0 1 1 1 1
  spline S146 degree 3 poles (-162.5373, -10.6443) (-162.3594, -10.9569) (-162.1044, -11.0381) (-161.7925, -10.9507) knots 0 0 0 0 1 1 1 1
  spline S147 degree 3 poles (-161.7925, -10.9507) (-161.4816, -10.8636) (-161.5975, -10.58) (-161.5931, -10.3749) knots 0 0 0 0 1 1 1 1
  spline S148 degree 3 poles (-161.5931, -10.3749) (-161.5787, -9.6978) (-161.5868, -9.0203) (-161.5845, -8.3429) knots 0 0 0 0 1 1 1 1
  spline S149 degree 3 poles (-161.5845, -8.3429) (-161.5822, -7.6653) (-161.5761, -7.6594) (-160.8742, -7.6552) knots 0 0 0 0 1 1 1 1
  spline S150 degree 3 poles (-160.8742, -7.6552) (-160.5094, -7.653) (-160.1427, -7.6783) (-159.7804, -7.6485) knots 0 0 0 0 1 1 1 1
  spline S151 degree 3 poles (-159.7804, -7.6485) (-159.2872, -7.608) (-159.11, -7.7892) (-159.1156, -8.2974) knots 0 0 0 0 1 1 1 1
  spline S152 degree 3 poles (-159.1156, -8.2974) (-159.1382, -10.3293) (-159.124, -12.3615) (-159.1234, -14.4458) knots 0 0 0 0 1 1 1 1
  spline S153 degree 3 poles (-163.4557, -13.4053) (-163.8868, -13.7171) (-164.1943, -14.1065) (-164.0824, -14.6696) knots 0 0 0 0 1 1 1 1
  spline S154 degree 3 poles (-164.0824, -14.6696) (-163.972, -15.2247) (-163.5649, -15.6177) (-163.0788, -15.6581) knots 0 0 0 0 1 1 1 1
  spline S155 degree 3 poles (-163.0788, -15.6581) (-162.7005, -15.6895) (-162.3178, -15.6674) (-161.9371, -15.6704) knots 0 0 0 0 1 1 1 1
  spline S156 degree 3 poles (-161.9371, -15.6704) (-161.702, -15.6723) (-161.5887, -15.5613) (-161.5901, -15.3225) knots 0 0 0 0 1 1 1 1
  spline S157 degree 3 poles (-161.5901, -15.3225) (-161.5936, -14.7339) (-161.591, -14.1453) (-161.5915, -13.5566) knots 0 0 0 0 1 1 1 1
  spline S158 degree 3 poles (-161.5915, -13.5566) (-161.5916, -13.3803) (-161.6535, -13.2359) (-161.8515, -13.2397) knots 0 0 0 0 1 1 1 1
  spline S159 degree 3 poles (-161.8515, -13.2397) (-162.3654, -13.2493) (-162.8913, -13.1275) (-163.4557, -13.4053) knots 0 0 0 0 1 1 1 1
  spline S160 degree 3 poles (-115.4182, -7.923) (-114.2216, -8.591) (-113.6158, -9.5597) (-113.6357, -10.9121) knots 0 0 0 0 1 1 1 1
  spline S161 degree 3 poles (-113.6357, -10.9121) (-113.6534, -12.1108) (-113.6484, -13.31) (-113.6384, -14.5089) knots 0 0 0 0 1 1 1 1
  spline S162 degree 3 poles (-113.6384, -14.5089) (-113.6175, -17.0213) (-115.4735, -18.4409) (-118.0256, -18.0831) knots 0 0 0 0 1 1 1 1
  spline S163 degree 3 poles (-118.0256, -18.0831) (-119.4859, -17.8784) (-120.4521, -17.0552) (-120.9221, -15.6518) knots 0 0 0 0 1 1 1 1
  spline S164 degree 3 poles (-120.9221, -15.6518) (-121.0015, -15.4147) (-121.0088, -15.1754) (-121.0082, -14.932) knots 0 0 0 0 1 1 1 1
  spline S165 degree 3 poles (-121.0082, -14.932) (-121.005, -13.6114) (-120.9996, -12.2908) (-120.9992, -10.9702) knots 0 0 0 0 1 1 1 1
  spline S166 degree 3 poles (-120.9992, -10.9702) (-120.9986, -9.2353) (-119.8918, -7.8765) (-118.1699, -7.6618) knots 0 0 0 0 1 1 1 1
  spline S167 degree 3 poles (-118.1699, -7.6618) (-117.2687, -7.5495) (-116.3287, -7.4908) (-115.4182, -7.923) knots 0 0 0 0 1 1 1 1
  spline S168 degree 3 poles (-116.9146, -9.9125) (-117.8292, -9.6604) (-118.4534, -10.1228) (-118.4706, -11.0553) knots 0 0 0 0 1 1 1 1
  spline S169 degree 3 poles (-118.4706, -11.0553) (-118.4832, -11.7322) (-118.5234, -12.4088) (-118.5267, -13.0857) knots 0 0 0 0 1 1 1 1
  spline S170 degree 3 poles (-118.5267, -13.0857) (-118.5298, -13.7096) (-118.5889, -14.3371) (-118.4624, -14.9569) knots 0 0 0 0 1 1 1 1
  spline S171 degree 3 poles (-118.4624, -14.9569) (-118.3464, -15.5247) (-117.8723, -15.8179) (-117.1465, -15.7733) knots 0 0 0 0 1 1 1 1
  spline S172 degree 3 poles (-117.1465, -15.7733) (-116.6079, -15.7402) (-116.2085, -15.3892) (-116.1995, -14.8565) knots 0 0 0 0 1 1 1 1
  spline S173 degree 3 poles (-116.1995, -14.8565) (-116.1769, -13.5192) (-116.1837, -12.1813) (-116.1872, -10.8437) knots 0 0 0 0 1 1 1 1
  spline S174 degree 3 poles (-116.1872, -10.8437) (-116.1883, -10.3947) (-116.4126, -10.0897) (-116.9146, -9.9125) knots 0 0 0 0 1 1 1 1
  spline S175 degree 3 poles (-156.3055, -7.6624) (-154.2232, -7.6592) (-152.1898, -7.6641) (-150.1564, -7.6541) knots 0 0 0 0 1 1 1 1
  spline S176 degree 3 poles (-150.1564, -7.6541) (-149.793, -7.6523) (-149.6196, -7.7526) (-149.6206, -8.1537) knots 0 0 0 0 1 1 1 1
  spline S177 degree 3 poles (-149.6206, -8.1537) (-149.6278, -11.2292) (-149.6266, -14.3049) (-149.608, -17.3803) knots 0 0 0 0 1 1 1 1
  spline S178 degree 3 poles (-149.608, -17.3803) (-149.6054, -17.8234) (-149.77, -17.9411) (-150.1863, -17.9378) knots 0 0 0 0 1 1 1 1
  spline S179 degree 3 poles (-150.1863, -17.9378) (-152.1674, -17.9219) (-154.1488, -17.9229) (-156.1299, -17.935) knots 0 0 0 0 1 1 1 1
  spline S180 degree 3 poles (-156.1299, -17.935) (-156.5289, -17.9374) (-156.6882, -17.8059) (-156.6806, -17.3935) knots 0 0 0 0 1 1 1 1
  spline S181 degree 3 poles (-156.6806, -17.3935) (-156.6418, -15.2993) (-156.9397, -15.6983) (-155.0051, -15.6644) knots 0 0 0 0 1 1 1 1
  spline S182 degree 3 poles (-155.0051, -15.6644) (-154.0367, -15.6475) (-153.0678, -15.6615) (-152.0964, -15.6615) knots 0 0 0 0 1 1 1 1
  spline S183 degree 3 poles (-152.0964, -15.6615) (-151.9724, -15.1549) (-152.005, -14.7043) (-152.004, -14.2562) knots 0 0 0 0 1 1 1 1
  spline S184 degree 3 poles (-152.004, -14.2562) (-152.0033, -13.8976) (-152.2589, -13.8971) (-152.5115, -13.8946) knots 0 0 0 0 1 1 1 1
  spline S185 degree 3 poles (-152.5115, -13.8946) (-153.6925, -13.8831) (-154.8739, -13.8519) (-156.0544, -13.8713) knots 0 0 0 0 1 1 1 1
  spline S186 degree 3 poles (-156.0544, -13.8713) (-156.5204, -13.8789) (-156.6559, -13.7108) (-156.6499, -13.2683) knots 0 0 0 0 1 1 1 1
  spline S187 degree 3 poles (-156.6499, -13.2683) (-156.6243, -11.3896) (-156.8256, -11.7342) (-155.1171, -11.7057) knots 0 0 0 0 1 1 1 1
  spline S188 degree 3 poles (-155.1171, -11.7057) (-154.2483, -11.6912) (-153.379, -11.6916) (-152.5103, -11.7082) knots 0 0 0 0 1 1 1 1
  spline S189 degree 3 poles (-152.5103, -11.7082) (-152.1322, -11.7154) (-151.9803, -11.5836) (-151.9907, -11.1939) knots 0 0 0 0 1 1 1 1
  spline S190 degree 3 poles (-151.9907, -11.1939) (-152.0322, -9.6338) (-151.7601, -9.9122) (-153.2627, -9.8899) knots 0 0 0 0 1 1 1 1
  spline S191 degree 3 poles (-153.2627, -9.8899) (-154.2184, -9.8757) (-155.1747, -9.8749) (-156.1302, -9.8929) knots 0 0 0 0 1 1 1 1
  spline S192 degree 3 poles (-156.1302, -9.8929) (-156.5283, -9.9003) (-156.7074, -9.7678) (-156.6841, -9.3529) knots 0 0 0 0 1 1 1 1
  spline S193 degree 3 poles (-156.6841, -9.3529) (-156.6606, -8.9371) (-156.6768, -8.519) (-156.6781, -8.1019) knots 0 0 0 0 1 1 1 1
  spline S194 degree 3 poles (-156.6781, -8.1019) (-156.6789, -7.8739) (-156.6385, -7.6803) (-156.3055, -7.6624) knots 0 0 0 0 1 1 1 1
  spline S195 degree 3 poles (-141.1188, -7.6505) (-140.3424, -7.6631) (-140.3405, -7.6631) (-140.3403, -8.367) knots 0 0 0 0 1 1 1 1
  spline S196 degree 3 poles (-140.3403, -8.367) (-140.3393, -11.3367) (-140.3491, -14.3066) (-140.3299, -17.2762) knots 0 0 0 0 1 1 1 1
  spline S197 degree 3 poles (-140.3299, -17.2762) (-140.3267, -17.7629) (-140.4492, -17.9503) (-140.966, -17.9344) knots 0 0 0 0 1 1 1 1
  spline S198 degree 3 poles (-140.966, -17.9344) (-142.1111, -17.8992) (-143.2581, -17.9294) (-144.4043, -17.9218) knots 0 0 0 0 1 1 1 1
  spline S199 degree 3 poles (-144.4043, -17.9218) (-145.9341, -17.9116) (-147.1858, -16.6651) (-147.1937, -15.1406) knots 0 0 0 0 1 1 1 1
  spline S200 degree 3 poles (-147.1937, -15.1406) (-147.2016, -13.6297) (-147.1314, -12.1152) (-147.2152, -10.6089) knots 0 0 0 0 1 1 1 1
  spline S201 degree 3 poles (-147.2152, -10.6089) (-147.2884, -9.2934) (-145.9538, -7.6562) (-144.1914, -7.6436) knots 0 0 0 0 1 1 1 1
  spline S202 degree 3 poles (-144.1914, -7.6436) (-143.1842, -7.6363) (-142.1768, -7.6475) (-141.1188, -7.6505) knots 0 0 0 0 1 1 1 1
  spline S203 degree 3 poles (-144.8293, -13.6624) (-144.8291, -13.9745) (-144.8298, -14.2867) (-144.8286, -14.5988) knots 0 0 0 0 1 1 1 1
  spline S204 degree 3 poles (-144.8286, -14.5988) (-144.8256, -15.4103) (-144.5937, -15.6476) (-143.7849, -15.6655) knots 0 0 0 0 1 1 1 1
  spline S205 degree 3 poles (-143.7849, -15.6655) (-143.6116, -15.6693) (-143.4366, -15.6527) (-143.265, -15.6705) knots 0 0 0 0 1 1 1 1
  spline S206 degree 3 poles (-143.265, -15.6705) (-142.832, -15.7154) (-142.6887, -15.5269) (-142.6944, -15.1001) knots 0 0 0 0 1 1 1 1
  spline S207 degree 3 poles (-142.6944, -15.1001) (-142.7126, -13.7479) (-142.6876, -12.3951) (-142.7021, -11.0427) knots 0 0 0 0 1 1 1 1
  spline S208 degree 3 poles (-142.7021, -11.0427) (-142.7162, -9.734) (-142.4498, -9.8847) (-143.9074, -9.8945) knots 0 0 0 0 1 1 1 1
  spline S209 degree 3 poles (-143.9074, -9.8945) (-144.4965, -9.8985) (-144.8244, -10.2601) (-144.8288, -10.8534) knots 0 0 0 0 1 1 1 1
  spline S210 degree 3 poles (-144.8288, -10.8534) (-144.8355, -11.7551) (-144.8298, -12.6568) (-144.8293, -13.6624) knots 0 0 0 0 1 1 1 1
  spline S211 degree 3 poles (-127.8249, -16.7371) (-127.8251, -17.9255) (-127.8251, -17.9255) (-128.9592, -17.9504) knots 0 0 0 0 1 1 1 1
  spline S212 degree 3 poles (-128.9592, -17.9504) (-130.1912, -17.9774) (-130.1911, -17.9774) (-130.1911, -16.7306) knots 0 0 0 0 1 1 1 1
  spline S213 degree 3 poles (-130.1911, -16.7306) (-130.1911, -14.7313) (-130.1914, -12.7321) (-130.1913, -10.7329) knots 0 0 0 0 1 1 1 1
  spline S214 degree 3 poles (-130.1913, -10.7329) (-130.1912, -8.8887) (-129.0298, -7.6616) (-127.1788, -7.5499) knots 0 0 0 0 1 1 1 1
  spline S215 degree 3 poles (-127.1788, -7.5499) (-126.0766, -7.4834) (-125.074, -7.7151) (-124.2491, -8.5061) knots 0 0 0 0 1 1 1 1
  spline S216 degree 3 poles (-124.2491, -8.5061) (-123.6685, -9.0628) (-123.3449, -9.7322) (-123.343, -10.5392) knots 0 0 0 0 1 1 1 1
  spline S217 degree 3 poles (-123.343, -10.5392) (-123.3376, -12.7992) (-123.3535, -15.0593) (-123.3304, -17.3191) knots 0 0 0 0 1 1 1 1
  spline S218 degree 3 poles (-123.3304, -17.3191) (-123.3256, -17.7927) (-123.485, -17.9532) (-123.9433, -17.982) knots 0 0 0 0 1 1 1 1
  spline S219 degree 3 poles (-123.9433, -17.982) (-125.7056, -18.0927) (-125.7044, -18.1037) (-125.705, -16.3572) knots 0 0 0 0 1 1 1 1
  spline S220 degree 3 poles (-125.705, -16.3572) (-125.7056, -14.5144) (-125.698, -12.6715) (-125.7126, -10.8289) knots 0 0 0 0 1 1 1 1
  spline S221 degree 3 poles (-125.7126, -10.8289) (-125.7192, -9.9981) (-126.5718, -9.5127) (-127.313, -9.8945) knots 0 0 0 0 1 1 1 1
  spline S222 degree 3 poles (-127.313, -9.8945) (-127.722, -10.1052) (-127.828, -10.4654) (-127.8267, -10.8967) knots 0 0 0 0 1 1 1 1
  spline S223 degree 3 poles (-127.8267, -10.8967) (-127.8206, -12.8264) (-127.8245, -14.7561) (-127.8249, -16.7371) knots 0 0 0 0 1 1 1 1
  spline S224 degree 3 poles (-132.7482, -10.4818) (-132.75, -12.7753) (-132.7657, -15.0168) (-132.7435, -17.2579) knots 0 0 0 0 1 1 1 1
  spline S225 degree 3 poles (-132.7435, -17.2579) (-132.7383, -17.7803) (-132.8927, -17.9882) (-133.4253, -17.939) knots 0 0 0 0 1 1 1 1
  spline S226 degree 3 poles (-133.4253, -17.939) (-133.7682, -17.9074) (-134.1196, -17.9451) (-134.4653, -17.974) knots 0 0 0 0 1 1 1 1
  spline S227 degree 3 poles (-134.4653, -17.974) (-134.9193, -18.012) (-135.111, -17.8685) (-135.1056, -17.3647) knots 0 0 0 0 1 1 1 1
  spline S228 degree 3 poles (-135.1056, -17.3647) (-135.0809, -15.0715) (-135.105, -12.7777) (-135.087, -10.4844) knots 0 0 0 0 1 1 1 1
  spline S229 degree 3 poles (-135.087, -10.4844) (-135.0835, -10.0389) (-135.2025, -9.8531) (-135.6728, -9.8782) knots 0 0 0 0 1 1 1 1
  spline S230 degree 3 poles (-135.6728, -9.8782) (-136.2965, -9.9115) (-136.9237, -9.873) (-137.5487, -9.8909) knots 0 0 0 0 1 1 1 1
  spline S231 degree 3 poles (-137.5487, -9.8909) (-137.9395, -9.902) (-138.1357, -9.7716) (-138.1138, -9.3541) knots 0 0 0 0 1 1 1 1
  spline S232 degree 3 poles (-138.1138, -9.3541) (-138.0939, -8.9728) (-138.0931, -8.589) (-138.1126, -8.2078) knots 0 0 0 0 1 1 1 1
  spline S233 degree 3 poles (-138.1126, -8.2078) (-138.1336, -7.7958) (-137.9432, -7.6546) (-137.5526, -7.6574) knots 0 0 0 0 1 1 1 1
  spline S234 degree 3 poles (-137.5526, -7.6574) (-136.1279, -7.6675) (-134.7031, -7.6675) (-133.2784, -7.661) knots 0 0 0 0 1 1 1 1
  spline S235 degree 3 poles (-133.2784, -7.661) (-132.9068, -7.6593) (-132.7408, -7.8081) (-132.7469, -8.1883) knots 0 0 0 0 1 1 1 1
  spline S236 degree 3 poles (-132.7469, -8.1883) (-132.759, -8.9352) (-132.7491, -9.6825) (-132.7482, -10.4818) knots 0 0 0 0 1 1 1 1
  spline S237 degree 3 poles (-142.8088, -3.0597) (-142.8094, -1.4299) (-142.8177, 0.1497) (-142.8038, 1.7291) knots 0 0 0 0 1 1 1 1
  spline S238 degree 3 poles (-142.8038, 1.7291) (-142.8011, 2.0286) (-142.964, 2.4246) (-142.5062, 2.5695) knots 0 0 0 0 1 1 1 1
  spline S239 degree 3 poles (-142.5062, 2.5695) (-141.9759, 2.7374) (-141.345, 2.5811) (-141.0994, 2.2053) knots 0 0 0 0 1 1 1 1
  spline S240 degree 3 poles (-141.0994, 2.2053) (-140.7199, 1.6246) (-140.3609, 1.0305) (-139.9905, 0.4438) knots 0 0 0 0 1 1 1 1
  spline S241 degree 3 poles (-139.9905, 0.4438) (-139.9191, 0.3308) (-139.8348, 0.226) (-139.6537, 0.1331) knots 0 0 0 0 1 1 1 1
  spline S242 degree 3 poles (-139.6537, 0.1331) (-139.6537, 0.713) (-139.66, 1.293) (-139.652, 1.8728) knots 0 0 0 0 1 1 1 1
  spline S243 degree 3 poles (-139.652, 1.8728) (-139.6431, 2.5164) (-139.5659, 2.5882) (-138.9292, 2.5953) knots 0 0 0 0 1 1 1 1
  spline S244 degree 3 poles (-138.9292, 2.5953) (-138.773, 2.597) (-138.6165, 2.5884) (-138.4606, 2.5959) knots 0 0 0 0 1 1 1 1
  spline S245 degree 3 poles (-138.4606, 2.5959) (-138.1412, 2.6111) (-137.963, 2.4724) (-137.962, 2.1449) knots 0 0 0 0 1 1 1 1
  spline S246 degree 3 poles (-137.962, 2.1449) (-137.9563, 0.253) (-137.953, -1.6389) (-137.9487, -3.5308) knots 0 0 0 0 1 1 1 1
  spline S247 degree 3 poles (-137.9487, -3.5308) (-137.9481, -3.7723) (-138.0511, -3.93) (-138.3018, -3.9642) knots 0 0 0 0 1 1 1 1
  spline S248 degree 3 poles (-138.3018, -3.9642) (-138.7177, -4.021) (-139.1384, -4.1053) (-139.4142, -3.649) knots 0 0 0 0 1 1 1 1
  spline S249 degree 3 poles (-139.4142, -3.649) (-139.836, -2.9512) (-140.2657, -2.258) (-140.6924, -1.5631) knots 0 0 0 0 1 1 1 1
  spline S250 degree 3 poles (-140.6924, -1.5631) (-140.7918, -1.4013) (-140.8928, -1.2404) (-141.0997, -1.0852) knots 0 0 0 0 1 1 1 1
  spline S251 degree 3 poles (-141.0997, -1.0852) (-141.0997, -1.7645) (-141.0992, -2.4439) (-141.0998, -3.1232) knots 0 0 0 0 1 1 1 1
  spline S252 degree 3 poles (-141.0998, -3.1232) (-141.1004, -3.9419) (-141.169, -4.0224) (-141.8637, -4.0234) knots 0 0 0 0 1 1 1 1
  spline S253 degree 3 poles (-141.8637, -4.0234) (-142.6938, -4.0246) (-142.7986, -3.9233) (-142.8088, -3.0597) knots 0 0 0 0 1 1 1 1
  spline S254 degree 3 poles (-148.635, 2.2773) (-148.1, 2.6445) (-147.5219, 2.6443) (-146.949, 2.6442) knots 0 0 0 0 1 1 1 1
  spline S255 degree 3 poles (-146.949, 2.6442) (-146.4806, 2.6442) (-146.0121, 2.6038) (-145.5436, 2.6037) knots 0 0 0 0 1 1 1 1
  spline S256 degree 3 poles (-145.5436, 2.6037) (-145.1988, 2.6036) (-145.0335, 2.4714) (-145.0344, 2.1117) knots 0 0 0 0 1 1 1 1
  spline S257 degree 3 poles (-145.0344, 2.1117) (-145.0393, 0.2357) (-145.0392, -1.6404) (-145.0296, -3.5164) knots 0 0 0 0 1 1 1 1
  spline S258 degree 3 poles (-145.0296, -3.5164) (-145.0277, -3.8733) (-145.1865, -4.0271) (-145.5265, -4.0268) knots 0 0 0 0 1 1 1 1
  spline S259 degree 3 poles (-145.5265, -4.0268) (-146.2212, -4.026) (-146.9184, -4.0604) (-147.6102, -4.0149) knots 0 0 0 0 1 1 1 1
  spline S260 degree 3 poles (-147.6102, -4.0149) (-148.698, -3.9432) (-149.4465, -3.11) (-149.4807, -1.9484) knots 0 0 0 0 1 1 1 1
  spline S261 degree 3 poles (-149.4807, -1.9484) (-149.5078, -1.0286) (-149.4955, -0.1072) (-149.4832, 0.8133) knots 0 0 0 0 1 1 1 1
  spline S262 degree 3 poles (-149.4832, 0.8133) (-149.4749, 1.4354) (-149.1385, 1.888) (-148.635, 2.2773) knots 0 0 0 0 1 1 1 1
  spline S263 degree 3 poles (-147.2644, 1.1474) (-147.5581, 1.0768) (-147.8164, 0.909) (-147.8272, 0.6081) knots 0 0 0 0 1 1 1 1
  spline S264 degree 3 poles (-147.8272, 0.6081) (-147.8577, -0.2401) (-147.8755, -1.0928) (-147.8182, -1.9384) knots 0 0 0 0 1 1 1 1
  spline S265 degree 3 poles (-147.8182, -1.9384) (-147.79, -2.3539) (-147.4039, -2.4358) (-147.0205, -2.4189) knots 0 0 0 0 1 1 1 1
  spline S266 degree 3 poles (-147.0205, -2.4189) (-146.622, -2.4013) (-146.6605, -2.1191) (-146.6594, -1.8605) knots 0 0 0 0 1 1 1 1
  spline S267 degree 3 poles (-146.6594, -1.8605) (-146.656, -1.0452) (-146.6691, -0.2296) (-146.6519, 0.5853) knots 0 0 0 0 1 1 1 1
  spline S268 degree 3 poles (-146.6519, 0.5853) (-146.6438, 0.9741) (-146.7711, 1.1858) (-147.2644, 1.1474) knots 0 0 0 0 1 1 1 1
  spline S269 degree 3 poles (-131.7115, -0.6647) (-131.9937, -1.6382) (-132.2463, -2.5757) (-132.431, -3.5302) knots 0 0 0 0 1 1 1 1
  spline S270 degree 3 poles (-132.431, -3.5302) (-132.4474, -3.6148) (-132.4536, -3.727) (-132.509, -3.7743) knots 0 0 0 0 1 1 1 1
  spline S271 degree 3 poles (-132.509, -3.7743) (-133.0204, -4.2107) (-133.6353, -3.9399) (-134.2023, -4.0017) knots 0 0 0 0 1 1 1 1
  spline S272 degree 3 poles (-134.2023, -4.0017) (-134.4987, -4.034) (-134.6206, -3.8268) (-134.6882, -3.5622) knots 0 0 0 0 1 1 1 1
  spline S273 degree 3 poles (-134.6882, -3.5622) (-135.1598, -1.7143) (-135.649, 0.1291) (-136.1074, 1.9802) knots 0 0 0 0 1 1 1 1
  spline S274 degree 3 poles (-136.1074, 1.9802) (-136.251, 2.5598) (-136.1298, 2.6727) (-135.5234, 2.6982) knots 0 0 0 0 1 1 1 1
  spline S275 degree 3 poles (-135.5234, 2.6982) (-135.4194, 2.7026) (-135.3104, 2.6945) (-135.2126, 2.7228) knots 0 0 0 0 1 1 1 1
  spline S276 degree 3 poles (-135.2126, 2.7228) (-134.754, 2.8558) (-134.5258, 2.6534) (-134.4258, 2.2206) knots 0 0 0 0 1 1 1 1
  spline S277 degree 3 poles (-134.4258, 2.2206) (-134.3699, 1.9786) (-134.4169, 1.6335) (-134.1036, 1.5695) knots 0 0 0 0 1 1 1 1
  spline S278 degree 3 poles (-134.1036, 1.5695) (-133.716, 1.4902) (-133.2992, 1.4869) (-132.9171, 1.6004) knots 0 0 0 0 1 1 1 1
  spline S279 degree 3 poles (-132.9171, 1.6004) (-132.708, 1.6625) (-132.7196, 1.9447) (-132.6601, 2.1413) knots 0 0 0 0 1 1 1 1
  spline S280 degree 3 poles (-132.6601, 2.1413) (-132.5126, 2.6293) (-131.4228, 2.9331) (-131.0576, 2.5803) knots 0 0 0 0 1 1 1 1
  spline S281 degree 3 poles (-131.0576, 2.5803) (-130.8836, 2.4121) (-130.9488, 2.1887) (-131.0006, 1.9901) knots 0 0 0 0 1 1 1 1
  spline S282 degree 3 poles (-131.0006, 1.9901) (-131.2283, 1.1173) (-131.4651, 0.2468) (-131.7115, -0.6647) knots 0 0 0 0 1 1 1 1
  spline S283 degree 3 poles (-133.7223, -0.6561) (-133.6446, -0.8196) (-133.6669, -1.0277) (-133.4782, -1.1792) knots 0 0 0 0 1 1 1 1
  spline S284 degree 3 poles (-133.4782, -1.1792) (-133.395, -0.787) (-133.2525, -0.4275) (-133.2976, -0.0354) knots 0 0 0 0 1 1 1 1
  spline S285 degree 3 poles (-133.2976, -0.0354) (-133.4825, 0.0363) (-133.6424, 0.063) (-133.8086, -0.0885) knots 0 0 0 0 1 1 1 1
  spline S286 degree 3 poles (-133.8086, -0.0885) (-133.7893, -0.247) (-133.7688, -0.4153) (-133.7223, -0.6561) knots 0 0 0 0 1 1 1 1
  spline S287 degree 3 poles (-122.9863, -0.484) (-123.5565, 0.3382) (-123.565, 1.1449) (-123.005, 1.9176) knots 0 0 0 0 1 1 1 1
  spline S288 degree 3 poles (-123.005, 1.9176) (-122.3878, 2.7694) (-121.479, 2.7876) (-120.5571, 2.6514) knots 0 0 0 0 1 1 1 1
  spline S289 degree 3 poles (-120.5571, 2.6514) (-120.0496, 2.5764) (-119.6158, 2.3156) (-119.2417, 1.9589) knots 0 0 0 0 1 1 1 1
  spline S290 degree 3 poles (-119.2417, 1.9589) (-119.0072, 1.7353) (-118.9887, 1.5176) (-119.2271, 1.2914) knots 0 0 0 0 1 1 1 1
  spline S291 degree 3 poles (-119.2271, 1.2914) (-119.3781, 1.1481) (-119.5358, 1.0119) (-119.6869, 0.8689) knots 0 0 0 0 1 1 1 1